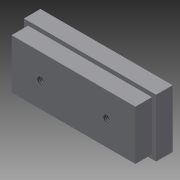
# Autodesk Inventor part: Endcaps
Saved by Autodesk Inventor 2014 (Build 180170000, 170)
## iProperties
Created: 2014-01-17
Part Number: Endcaps
Material: Generic
Document SubType Name: Modeling
Designer: james.eddlestone
Density: 1 g/cm^3
Appearance: Default
Author: james.eddlestone
Autodesk Inventor part; units mm, degrees
ref_plane "YZ Plane" through (0, 0, 0) normal (1, 0, 0) x (0, 1, 0)
ref_plane "XZ Plane" through (0, 0, 0) normal (0, 1, 0) x (-1, 0, 0)
ref_plane "XY Plane" through (0, 0, 0) normal (0, 0, 1) x (1, 0, 0)
sketch "Sketch1" plane through (0, 0, 0) normal (0, 0, 1) x (1, 0, 0)
  line L0 (0, 0) -> (101.6, 0)
  line L1 (101.6, 0) -> (101.6, 44.45)
  line L2 (101.6, 44.45) -> (0, 44.45)
  line L3 (0, 44.45) -> (0, 0)
  dimension "d0" = 101.6
  dimension "d1" = 44.45
  constraints: 8 end point, 2 parallel, 1 horizontal, 1 perpendicular
  measures "d0" distance of L2.end L1.end
  measures "d1" distance of L1.end L0.end
extrude "Extrusion1" add sketch "Sketch1" along normal blind 25.4
sketch "Sketch2" plane through (0, 0, 25.4) normal (0, 0, 1) x (1, 0, 0)
  line L0 (0, 0) -> (101.6, 0) projected
  line L1 (101.6, 0) -> (101.6, 44.45) projected
  line L2 (101.6, 44.45) -> (0, 44.45) projected
  line L3 (0, 44.45) -> (0, 0) projected
  line L4 (3.175, 41.275) -> (98.425, 41.275)
  line L5 (98.425, 41.275) -> (98.425, 3.175)
  line L6 (98.425, 3.175) -> (3.175, 3.175)
  line L7 (3.175, 3.175) -> (3.175, 41.275)
  dimension "d4" = 3.175
  constraints: 8 end point, 3 other
  measures "d4" distance between parallel lines of L2 L4
extrude "Extrusion2" cut sketch "Sketch2" against normal blind 12.7
sketch "Sketch3" plane through (0, 0, 0) normal (0, 0, -1) x (-1, 0, 0)
  line L0 (0, 44.45) -> (0, 0) projected
  line L1 (-101.6, 44.45) -> (0, 44.45) projected
  line L2 (-101.6, 0) -> (-101.6, 44.45) projected
  point P0 (-76.2, 22.225)
  point P1 (-25.4, 22.225)
  dimension "d7" = 50.8
  dimension "d8" = 25.4
  dimension "d9" = 25.4
  dimension "d10" = 22.225
  measures "d7" distance of point (-25.4, 22.225) point (-76.2, 22.225)
  measures "d8" distance from line of L2 point (-76.2, 22.225)
  measures "d9" distance from line of L0 point (-25.4, 22.225)
  measures "d10" distance from line of point (-25.4, 22.225) L1
hole "Hole1" at (76.2, 22.225, 0) at (25.4, 22.225, 0) direction (0, 0, 1) diameter 4.9784 end through all thread size "1/4-20 UNC" class "2B" standard "ANSI Unified Screw Threads"
body "Solid1"
